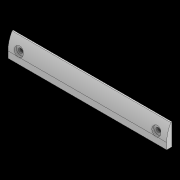
# Autodesk Inventor part: top_140mm_2
Saved by Autodesk Inventor 2022 (Build 260153000, 153)
## iProperties
Created: 2022-10-14
Part Number: top_140mm_2
Material: 一般
Document SubType Name: Modeling
Designer: numai
Density: 1 g/cm^3
Appearance: 既定
Author: numai
Autodesk Inventor part; units mm, degrees
ref_plane "YZ Plane" through (0, 0, 0) normal (1, 0, 0) x (0, 1, 0)
ref_plane "XZ Plane" through (0, 0, 0) normal (0, 1, 0) x (-1, 0, 0)
ref_plane "XY Plane" through (0, 0, 0) normal (0, 0, 1) x (1, 0, 0)
sketch "スケッチ1" plane through (0, 0, 0) normal (0, 0, 1) x (1, 0, 0)
  line L0 (-75, 20.5) -> (75, 20.5)
  line L1 (75, 20.5) -> (75, 0)
  line L2 (75, 0) -> (-75, 0)
  line L3 (-75, 0) -> (-75, 20.5)
  circle A0 centre (-65, 10.25) radius 4.25
  circle A1 centre (65, 10.25) radius 4.25
  point P0 (0, 0)
  point P1 (0, 0)
  dimension "d0" = 20.5
  dimension "d1" = 150
  dimension "d2" = 10.25
  dimension "d3" = 130
  dimension "d4" = 10
  dimension "d5" = 8.5
  constraints: 8 end point, 2 centre point, 2 parallel, 1 coincident, 1 equal radius, 1 horizontal, 1 horizontal alignment, 1 midpoint, 1 perpendicular
  measures "d0" distance of L0.end L1.end
  measures "d1" distance of L0.start L0.end
  measures "d2" distance from line of L2 A0.centre
  measures "d3" distance of A1.centre A0.centre
  measures "d4" distance from line of L1 A1.centre
  measures "d5" diameter of A1
extrude "押し出し1" add sketch "スケッチ1" along normal blind 5
sketch "スケッチ3" plane through (75, 0, 0) normal (1, 0, 0) x (0, 0, -1)
  line L0 (0, 0) -> (0, 20.5) construction
  line L1 (0, 20.5) -> (-5, 20.5) construction
  line L2 (-5, 0) -> (-5, 20.5) construction
  line L3 (0, 0) -> (-5, 0) construction
  line L4 (0, 20.5) -> (-5, 20.5) projected
  arc A0 (-1.2, 20.5) -> (-5, 6) centre (24.5645, 6) ccw
  line L5 (-5, 0) -> (-5, 20.5) projected
  line L6 (-1.2, 20.5) -> (-5, 13.7479) construction
  line L7 (-1.2, 20.5) -> (-5, 20.5)
  line L8 (-5, 6) -> (-5, 20.5)
  point P0 (0, 0)
  dimension "d12" = 1.2
  dimension "d13" = 6
  constraints: 6 end point, 3 point on line, 3 tangent, 2 point on circle, 1 centre point, 1 collinear, 1 perpendicular
  measures "d12" distance of L0.end L6.start
  measures "d13" distance from line of L3 L8.start
extrude "押し出し3" cut sketch "スケッチ3" against normal through all
sketch "スケッチ4" plane through (0, 0, 0) normal (0, 0, -1) x (-1, 0, 0)
  circle A0 centre (-65, 10.25) radius 4.25 projected
  circle A1 centre (65, 10.25) radius 4.25 projected
  circle A2 centre (-65, 10.25) radius 2.15
  circle A3 centre (65, 10.25) radius 2.15
  point P0 (0, 0)
  dimension "d16" = 4.3
  constraints: 2 centre point, 2 coincident, 1 equal radius
  measures "d16" diameter of A2
extrude "押し出し4" add sketch "スケッチ4" against normal blind 3
equation "\"d2\" = 0.5 * d0"
equation "\"d4\" = -0.5 * d3 + 0.5 * d1"
